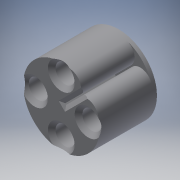
# Autodesk Inventor part: Sample_holder_simple
Saved by Autodesk Inventor 2019 (Build 230136000, 136)
## iProperties
Created: 2021-10-14
Part Number: Sample_holder_simple
Material: Generic
Document SubType Name: Modeling
Designer: Pokick
Density: 1 g/cm^3
Appearance: Default
Author: Pokick
Autodesk Inventor part; units mm, degrees
ref_plane "YZ Plane" through (0, 0, 0) normal (1, 0, 0) x (0, 1, 0)
ref_plane "XZ Plane" through (0, 0, 0) normal (0, 1, 0) x (-1, 0, 0)
ref_plane "XY Plane" through (0, 0, 0) normal (0, 0, 1) x (1, 0, 0)
sketch "Sketch1" plane through (0, 0, 0) normal (0, 0, 1) x (1, 0, 0)
  circle A0 centre (0, 0) radius 10
  circle A1 centre (0, 0) radius 7 construction
  line L0 (0, 0) -> (0, 10) construction
  circle A2 centre (0, 7) radius 1.5
  line L1 (0, 0) -> (-10, 0) construction
  circle A3 centre (-7, 0) radius 1.5
  line L2 (0, 0) -> (0, -10) construction
  circle A4 centre (0, -7) radius 1.5
  line L3 (0, 0) -> (10, 0) construction
  circle A5 centre (7, 0) radius 1.5
  dimension "d0" = 20
  dimension "d1" = 14
  dimension "d2" = 3
  dimension "d5" = 360
  constraints: 8 end point, 4 centre point, 4 point on line, 2 coincident, 2 vertical alignment, 1 vertical, 25 other
  measures "d2" diameter of A2
extrude "Extrusion1" add sketch "Sketch1" along normal blind 15
sketch "Sketch2" plane through (0, 0, 15) normal (0, 0, 1) x (1, 0, 0)
  circle A0 centre (0, 0) radius 7 construction
  line L0 (0, 0) -> (0, 7) construction
  line L1 (0, 0) -> (7, 0) construction
  line L2 (0, 0) -> (7, 0) construction
  line L3 (7, 0) -> (7, 7) construction
  line L4 (7, 7) -> (0, 7) construction
  line L5 (0, 7) -> (0, 0) construction
  circle A1 centre (0, 0) radius 0.25 construction
  line L6 (0, 0.25) -> (0.25, 0)
  line L7 (0.25, 0) -> (7.3211, 7.0711)
  line L8 (7.3211, 7.0711) -> (7.0711, 7.3211)
  line L9 (7.0711, 7.3211) -> (0, 0.25)
  circle A2 centre (7, 0) radius 2.5
  circle A3 centre (0, 0) radius 10 construction
  circle A4 centre (0, 7) radius 2.5
  circle A5 centre (-7, 0) radius 2.5
  circle A6 centre (0, -7) radius 2.5
  dimension "d9" = 14
  dimension "d10" = 7
  dimension "d11" = 7
  dimension "d12" = 0.5
  dimension "d13" = 10
  dimension "d14" = 5
  dimension "d15" = 20
  dimension "d18" = 360
  constraints: 20 end point, 7 centre point, 4 coincident, 4 parallel, 4 point on circle, 2 horizontal, 2 perpendicular, 2 point on line, 1 vertical, 9 other
  measures "d9" diameter of A0
  measures "d10" distance of L4.end L3.end
  measures "d11" distance of L3.end L2.end
  measures "d12" diameter of A1
  measures "d13" distance of L7.end L6.end
  measures "d14" diameter of A2
  measures "d15" diameter of A3
extrude "Extrusion2" cut sketch "Sketch2" against normal blind 14
chamfer "Chamfer1" distance 1 angle 45 4 edges at (-2.5, -7, 15) (-2.5, 7, 15) (4.5, 0, 15) (-9.5, 0, 15)
chamfer "Chamfer2" distance 1 angle 45 2 edges at (3.4725, 3.7225, 15) (3.7225, 3.4725, 15)
fillet "Fillet1" radius 3 2 edges at (6.945, 7.195, 7.5) (7.195, 6.945, 7.5)
body "Solid1"
